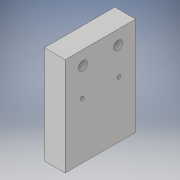
# Autodesk Inventor part: magMount
Saved by Autodesk Inventor 2017 (Build 210142000, 142)
## iProperties
Created: 2017-03-21
Part Number: magMount
Material: Generic
Document SubType Name: Modeling
Designer: Naga
Density: 1 g/cm^3
Appearance: Default
Author: Naga
Autodesk Inventor part; units mm, degrees
ref_plane "YZ Plane" through (0, 0, 0) normal (1, 0, 0) x (0, 1, 0)
ref_plane "XZ Plane" through (0, 0, 0) normal (0, 1, 0) x (-1, 0, 0)
ref_plane "XY Plane" through (0, 0, 0) normal (0, 0, 1) x (1, 0, 0)
sketch "Sketch1" plane through (0, 0, 0) normal (1, 0, 0) x (0, 1, 0)
  line L0 (0, 0) -> (10, 0)
  line L1 (10, 0) -> (10, -25.4)
  line L2 (10, -25.4) -> (0, -25.4)
  line L3 (0, -25.4) -> (0, 0)
  line L4 (5, 0) -> (5, -25.4) construction
  line L5 (10, 0) -> (0, 0)
  line L6 (0, 0) -> (0, -6.35)
  line L7 (0, -6.35) -> (10, -6.35) construction
  line L8 (10, -6.35) -> (10, 0)
  line L9 (10, -25.4) -> (0, -25.4)
  line L10 (0, -25.4) -> (0, -19.05)
  line L11 (0, -19.05) -> (10, -19.05) construction
  line L12 (10, -19.05) -> (10, -25.4)
  circle A0 centre (5, -6.35) radius 1.5875
  circle A1 centre (5, -19.05) radius 1.5875
  line L13 (0, -12.7) -> (-12.7, -12.7)
  line L14 (-3.302, -21.59) -> (-22.098, -21.59)
  line L15 (-22.098, -21.59) -> (-22.098, -3.81)
  line L16 (-22.098, -3.81) -> (-3.302, -3.81)
  line L17 (-3.302, -3.81) -> (-3.302, -21.59)
  line L18 (-3.302, -21.59) -> (-22.098, -3.81) construction
  line L19 (-22.098, -21.59) -> (-3.302, -3.81) construction
  line L20 (-22.098, -3.81) -> (-5.08, -3.81)
  line L21 (-5.08, -3.81) -> (-5.08, -6.096)
  circle A2 centre (-5.08, -6.096) radius 0.635
  circle A3 centre (-5.08, -19.304) radius 0.635
  line L22 (-25.4, 0) -> (0, 0)
  line L23 (0, 0) -> (0, -25.4)
  line L24 (0, -25.4) -> (-25.4, -25.4)
  line L25 (-25.4, -25.4) -> (-25.4, 0)
  line L26 (-25.4, 0) -> (0, -25.4) construction
  line L27 (0, 0) -> (-25.4, -25.4) construction
  dimension "d0" = 10
  dimension "d1" = 25.4
  dimension "d2" = 6.35
  dimension "d3" = 6.35
  dimension "d4" = 3.175
  dimension "d5" = 3.175
  dimension "d6" = 12.7
  dimension "d7" = 18.796
  dimension "d8" = 17.78
  dimension "d9" = 17.018
  dimension "d10" = 2.286
  dimension "d11" = 1.27
  constraints: 56 end point, 10 parallel, 9 midpoint, 6 horizontal, 6 perpendicular, 4 centre point, 3 point on line, 1 coincident, 1 symmetric about line, 1 other
  measures "d0" distance of L1.end L2.end
  measures "d1" distance of L0.end L1.end
  measures "d2" distance of L6.end L5.end
  measures "d3" distance of L9.end L10.end
  measures "d4" diameter of A0
  measures "d5" diameter of A1
  measures "d6" distance of L13.start L13.end
  measures "d7" distance of L15.end L16.end
  measures "d8" distance of L14.end L15.end
  measures "d9" distance of L15.end L20.end
  measures "d10" distance of L20.end L21.end
  measures "d11" diameter of A2
extrude "Extrusion1" add sketch "Sketch1" along normal blind 7.5 contours L0 L1 L2 L3 | L3 L24 L25 L22 | L14 L15 L16 L17
body "Solid1"
